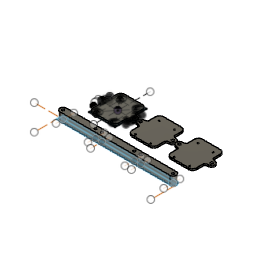
Multi FS40 Bracket v19 (Autodesk Fusion 360 design; units mm, degrees)
Autodesk Fusion 360 part; units mm, degrees
sketch "Schizzo1" plane through (0, 0, 0) normal (0, 0, 1) x (1, 0, 0)
  line L0 (32, -39) -> (-32, -39)
  line L1 (-32, -39) -> (-32, 39)
  line L2 (-32, 39) -> (32, 39)
  line L3 (32, 39) -> (32, -39)
  line L4 (32, -39) -> (-32, 39) construction
  line L5 (-32, -39) -> (32, 39) construction
  line L6 (-19.25, 24.7) -> (19.25, 24.7) construction
  line L7 (19.25, 24.7) -> (19.25, -33.8) construction
  line L8 (19.25, -33.8) -> (-19.25, -33.8) construction
  line L9 (-19.25, -33.8) -> (-19.25, 24.7) construction
  circle A0 centre (-19.25, 24.7) radius 1.7
  line L10 (0, 0) -> (0, 80) construction
  line L11 (0, 0) -> (0, -60) construction
  line L12 (-32, 0) -> (32, 0) construction
  circle A1 centre (-19.25, -33.8) radius 1.7
  circle A2 centre (19.25, -33.8) radius 1.7
  circle A3 centre (19.25, 24.7) radius 1.7
  line L13 (-32, 0) -> (-48, 0) construction
  line L14 (-40, 20.7498) -> (-40, -19.8726) construction
  circle A4 centre (-40, 0) radius 8
  line L15 (-40, -8) -> (-46, -8) construction
  line L16 (-46, -11.1) -> (-32, -11.1) construction
  arc A5 (-32, -11.1) -> (-40, -8) centre (-40, -19.8726) ccw
  arc A6 (-40, 8) -> (-32, 11.1) centre (-40, 19.8726) ccw
  circle A7 centre (40, 0) radius 8
  arc A8 (32, 11.1) -> (40, 8) centre (40, 19.8726) ccw
  arc A9 (40, -8) -> (32, -11.1) centre (40, -19.8726) ccw
  line L17 (-56.7434, -78.6442) -> (226.9, -78.6442)
  line L18 (226.9, -78.6442) -> (226.9, -94.6442)
  line L19 (226.9, -94.6442) -> (-56.7434, -94.6442)
  line L20 (-56.7434, -94.6442) -> (-56.7434, -78.6442)
  circle A10 centre (-48.7434, -86.6442) radius 8
  line L21 (-48.7434, -60) -> (-48.7434, -104.1406) construction
  circle A11 centre (-48.7434, -86.6442) radius 2.9
  line L22 (31.2566, -65) -> (31.2566, -105) construction
  line L23 (226.9, -86.6442) -> (-120, -86.6442) construction
  circle A12 centre (31.2566, -86.6442) radius 2.9
  line L24 (47.4566, -68.4362) -> (47.4566, -114.7306) construction
  circle A13 centre (47.4566, -86.6442) radius 2.9
  line L25 (127.4566, -70) -> (127.4566, -110) construction
  circle A14 centre (127.4566, -86.6442) radius 2.9
  line L26 (143.6566, -70) -> (143.6566, -110) construction
  line L27 (223.6566, -70) -> (223.6566, -110) construction
  circle A15 centre (143.6566, -86.6442) radius 2.9
  circle A16 centre (223.6566, -86.6442) radius 2.9
  circle A17 centre (223.6566, -86.6442) radius 8
  line L28 (-56.7434, -86.6442) -> (231.6566, -86.6442)
  line L29 (231.6566, -86.6442) -> (-56.7434, -86.6442)
  line L30 (-56.7434, -86.6442) -> (-56.7434, -150) construction
  line L31 (231.6566, -86.6442) -> (231.6566, -150) construction
  circle A18 centre (-40, 0) radius 3.1
  circle A19 centre (40, 0) radius 3.1
  circle A20 centre (-22, -29) radius 10
  circle A21 centre (22, -29) radius 10
  circle A22 centre (-22, 29) radius 10
  circle A23 centre (22, 29) radius 10
  dimension "d1" = 64
  dimension "d2" = 78
  dimension "d3" = 33.8
  dimension "d5" = 58.5
  dimension "d6" = 19.25
  dimension "d7" = 38.5
  dimension "d8" = 3.4
  dimension "d9" = 3.4
  dimension "d17" = 8
  dimension "d18" = 16
  dimension "d19" = 3.1
  dimension "d20" = 80
  dimension "d21" = 16
  dimension "d22" = 8
  dimension "d23" = 5.8
  dimension "d24" = 80
  dimension "d25" = 5.8
  dimension "d28" = 96.2
  dimension "d29" = 5.8
  dimension "d30" = 80
  dimension "d32" = 5.8
  dimension "d33" = 96.2
  dimension "d34" = 80
  dimension "d35" = 5.8
  dimension "d36" = 5.8
  dimension "d39" = 6.2
  dimension "d87" = 10
  dimension "d88" = 288.4
  constraint horizontal L0
  constraint perpendicular L0 L1
  constraint parallel L0 L2
  constraint parallel L1 L3
  constraint coincident L4 L10.start
  constraint coincident L5 L10.start
  constraint coincident L10.start L11.start
  constraint horizontal L6
  constraint vertical L7
  constraint horizontal L8
  constraint vertical L9
  constraint coincident L6.start L9.end
  constraint perpendicular L2 L10
  constraint perpendicular L0 L11
  constraint midpoint L1 L12.start
  constraint midpoint L3 L12.end
  constraint coincident L8.end L9.start
  constraint symmetric A0 L11 A3
  constraint symmetric L11 A1 A2
  constraint perpendicular L1 L13
  constraint vertical L14
  constraint coincident A4 L15.start
  constraint coincident L14 L15.start
  constraint tangent A4 L15
  constraint horizontal L16
  constraint coincident L1 L16.end
  constraint coincident L14 A5.centre
  constraint symmetric L13 L15.start A6.start
  constraint symmetric L13 L16.end A6.end
  constraint symmetric L13 A5 A6
  constraint symmetric L10 A4 A7
  constraint symmetric L10 L15.start A9.start
  constraint symmetric L10 L16.end A9.end
  constraint symmetric L10 A5 A9
  constraint symmetric L10 A6.end A8.start
  constraint symmetric L10 A6.start A8.end
  constraint symmetric L10 A6 A8
  constraint horizontal L17
  constraint vertical L18
  constraint horizontal L19
  constraint vertical L20
  constraint tangent L20 A10
  constraint tangent L19 A10
  constraint perpendicular L17 L21
  constraint coincident A10.centre L21
  constraint concentric A10 A11
  constraint perpendicular L19 L22
  constraint midpoint L18 L23.start
  constraint perpendicular L21 L23
  constraint coincident L22 A12.centre
  constraint coincident L23 A12.centre
  constraint perpendicular L19 L24
  constraint coincident L24 A13.centre
  constraint coincident L23 A13.centre
  constraint perpendicular L19 L25
  constraint coincident L25 A14.centre
  constraint coincident L23 A14.centre
  constraint perpendicular L19 L26
  constraint perpendicular L19 L27
  constraint coincident L26 A15.centre
  constraint coincident L23 A15.centre
  constraint coincident L27 A16.centre
  constraint coincident L23 A16.centre
  constraint concentric A16 A17
  constraint tangent L17 A17
  constraint midpoint L20 L28.start
  constraint coincident A17 L28.end
  constraint coincident L23 L28.end
  constraint tangent A10 L30
  constraint perpendicular L28 L30
  constraint tangent A17 L31
  constraint coincident L14.end A5.centre
  constraint coincident L13 A4.centre
  constraint concentric A4 A18
  constraint symmetric L10 A18 A19
  constraint tangent L1 A20
  constraint tangent L0 A20
  constraint symmetric L11 A20 A21
  constraint symmetric L12 A20 A22
  constraint symmetric L12 A21 A23
  measures "d1" distance of L1.end L2.end
  measures "d2" distance of L0.end L1.end
  measures "d3" distance of L10.start L8
  measures "d5" distance of L6 L8
  measures "d6" distance of L10.start L9
  measures "d7" distance of L7 L9
  measures "d8" diameter of A0
  measures "d9" diameter of A1
  measures "d17" distance of L1 L14.start
  measures "d18" diameter of A4
  measures "d19" distance of L15 L16
  measures "d20" distance of L14 A7.centre
  measures "d21" distance of L17.start L19.end
  measures "d22" radius of A10
  measures "d23" diameter of A11
  measures "d24" distance of L21 L22
  measures "d25" diameter of A12
  measures "d28" distance of A10.centre L24
  measures "d29" diameter of A13
  measures "d30" distance of L24 L25
  measures "d32" diameter of A14
  measures "d33" distance of L24 L26.end
  measures "d34" distance of L26 L27
  measures "d35" diameter of A15
  measures "d36" diameter of A16
  measures "d39" diameter of A18
  measures "d87" radius of A20
  measures "d88" distance of L30 L31
extrude "Estrusione1" add sketch "Schizzo1" along normal blind 4 contours L0 L1 L2 L3 A20 A21 A22 A23 | A21 | A20 | L3 A7 A9 | L3 A7 A8 | A7 | L1 A4 A5 | L1 A4 A6 | A4 | A23 | A22 makes body 1
pattern_linear "Serie R1" count 1 spacing 0 along (0, 1, 0) count 3 spacing 96.2 along (1, 0, 0) of bodies 1 makes body 2 at (102.3333, 0.3426, 0) makes body 3 at (198.5333, 0.3426, 0)
extrude "Estrusione2" add sketch "Schizzo1" along normal blind 20 separate body contours L17 A10 A12 A13 A14 A15 A17 L28 L29 | A10 A11 L28 L29 | A10 A11 L28 L29 | L18 A16 A17 L28 L29 | L19 A10 A12 A13 A14 A15 A17 L28 L29 | L18 A17 L28 L29 | L18 A16 A17 L28 L29 | L18 A17 L28 L29 makes body 4
sketch "Schizzo2" plane through (0, 0, 0) normal (0, 0, 1) x (1, 0, 0)
  line L0 (-157.1405, -8.0769) -> (-137.1405, -8.0769)
  line L1 (-137.1405, -8.0769) -> (-137.1405, -3.6769)
  line L2 (-137.1405, -3.6769) -> (-157.1405, -3.6769)
  line L3 (-157.1405, -3.6769) -> (-157.1405, -8.0769)
  line L4 (-157.1405, -5.8769) -> (-137.1405, -5.8769) construction
  line L5 (-147.1405, -3.6769) -> (-147.1405, -8.0769) construction
  line L6 (-141.6405, -8.0769) -> (-152.6405, -8.0769)
  line L7 (-152.6405, -8.0769) -> (-152.6405, -3.6769)
  line L8 (-152.6405, -3.6769) -> (-141.6405, -3.6769)
  line L9 (-141.6405, -3.6769) -> (-141.6405, -8.0769)
  line L10 (-141.6405, -8.0769) -> (-152.6405, -3.6769) construction
  line L11 (-152.6405, -8.0769) -> (-141.6405, -3.6769) construction
  line L12 (-141.6405, -6.6769) -> (-152.6405, -6.6769)
  line L13 (-152.6405, -6.6769) -> (-152.6405, -5.0769)
  line L14 (-152.6405, -5.0769) -> (-141.6405, -5.0769)
  line L15 (-141.6405, -5.0769) -> (-141.6405, -6.6769)
  line L16 (-141.6405, -6.6769) -> (-152.6405, -5.0769) construction
  line L17 (-152.6405, -6.6769) -> (-141.6405, -5.0769) construction
  line L18 (-157.1405, 2.1231) -> (-45.1405, 2.1231)
  line L19 (-45.1405, 2.1231) -> (-45.1405, -13.8769)
  line L20 (-45.1405, -13.8769) -> (-157.1405, -13.8769)
  line L21 (-157.1405, -13.8769) -> (-157.1405, 2.1231)
  line L22 (-101.1405, 2.1231) -> (-101.1405, -35) construction
  line L23 (-49.6405, -3.6769) -> (-60.6405, -3.6769)
  line L24 (-60.6405, -3.6769) -> (-60.6405, -8.0769)
  line L25 (-49.6405, -5.0769) -> (-60.6405, -5.0769)
  line L26 (-49.6405, -8.0769) -> (-49.6405, -3.6769)
  line L27 (-60.6405, -6.6769) -> (-49.6405, -6.6769)
  line L28 (-60.6405, -8.0769) -> (-49.6405, -8.0769)
  line L29 (-152.6405, -5.8769) -> (-36.8883, -5.8769) construction
  line L30 (-96.1405, 2.1231) -> (-96.1405, -17) construction
  circle A0 centre (-96.1405, -5.8769) radius 5
  point P0 (-147.1405, -5.8769)
  point P1 (-147.1405, -5.8769)
  dimension "d40" = 20
  dimension "d41" = 4.4
  dimension "d42" = 11
  dimension "d43" = 4.4
  dimension "d44" = 11
  dimension "d45" = 1.6
  dimension "d50" = 112
  dimension "d51" = 8
  dimension "d52" = 16
  dimension "d69" = 103
  dimension "d70" = 1.4
  dimension "d74" = 5
  constraint horizontal L0
  constraint vertical L1
  constraint horizontal L2
  constraint vertical L3
  constraint midpoint L3 L4.start
  constraint midpoint L1 L4.end
  constraint midpoint L2 L5.start
  constraint midpoint L0 L5.end
  constraint horizontal L6
  constraint perpendicular L6 L7
  constraint parallel L6 L8
  constraint parallel L7 L9
  constraint coincident L10 P1
  constraint coincident L11 P1
  constraint midpoint L5 P1
  constraint horizontal L12
  constraint perpendicular L12 L13
  constraint parallel L12 L14
  constraint parallel L13 L15
  constraint coincident L16 P1
  constraint coincident L17 P1
  constraint coincident P1 P0
  constraint horizontal L18
  constraint vertical L19
  constraint horizontal L20
  constraint vertical L21
  constraint collinear L3 L21
  constraint midpoint L18 L22.start
  constraint perpendicular L20 L22
  constraint symmetric L6.start L22 L24.end
  constraint symmetric L6.end L22 L26.start
  constraint symmetric L7.end L22 L23.start
  constraint symmetric L8.end L22 L23.end
  constraint symmetric L12.start L22 L27.start
  constraint symmetric L12.end L22 L27.end
  constraint symmetric L13.end L22 L25.start
  constraint symmetric L14.end L22 L25.end
  constraint midpoint L7 L29.start
  constraint perpendicular L1 L29
  constraint perpendicular L18 L30
  constraint coincident L18 L30.start
  constraint coincident L30 A0.centre
  constraint coincident L29 A0.centre
  constraint tangent L22 A0
  measures "d40" distance of L1 L3
  measures "d41" distance of L0 L2
  measures "d42" distance of L7.end L8.end
  measures "d43" distance of L6.end L7.end
  measures "d44" distance of L13.end L14.end
  measures "d45" distance of L12.end L13.end
  measures "d50" distance of L19 L21
  measures "d51" distance of L4.start L18.start
  measures "d52" distance of L18 L20
  measures "d69" distance of L7 L26
  measures "d70" distance of L8.end L14
  measures "d74" distance of L22 L30
extrude "Estrusione3" add sketch "Schizzo2" along normal blind 3 separate body contours L0 L6 L7 L9 L12 | L2 L7 L8 L9 L14 | L23 L24 L25 L26 | L24 L26 L27 L28 makes body 5 at (-148.9738, -8.0769, 1) makes body 6 at (-145.3071, -3.6769, 1) makes body 7 at (-56.9738, -8.0769, 1) makes body 8 at (-53.3071, -5.0769, 1)
extrude "Estrusione4" add sketch "Schizzo2" against normal blind 20 separate body contours L0 L2 L3 L7 L13 L21 | L0 L1 L2 L6 L8 L18 L19 L20 L21 | L0 L6 L7 L9 L12 | L0 L1 L2 L9 L15 | L7 L9 L12 L13 L14 L15 | L2 L7 L8 L9 L14 | L23 L24 L25 L26 | L24 L25 L26 L27 | L24 L26 L27 L28 | A0 makes body 9
combine "Combina1" operation add target body 6 tool bodies 9
combine "Combina2" operation add target body 5 tool bodies 6
sketch "Schizzo3" plane through (-152.6405, 0, 0) normal (-1, 0, 0) x (0, -1, 0)
  line L0 (3.6769, 0) -> (5.0769, 0)
  line L1 (5.0769, 0) -> (5.0769, 3)
  line L2 (5.0769, 3) -> (3.6769, 3)
  line L3 (3.6769, 3) -> (3.6769, 0)
sketch "Schizzo5" plane through (-152.6405, -5.3769, 2.25) normal (-1, 0, 0) x (0, -1, 0)
  line L0 (0, 0.7406) -> (0, 4.484) construction
  line L1 (1, 0.7406) -> (1, 4.4786) construction
  line L2 (0, 0.7406) -> (1, 0.7406) construction
  line L3 (0.5, 0.7406) -> (0.5, 3.1) construction
  line L4 (0, 0.7406) -> (-2.9121, 0.7406) construction
  line L5 (0, 0.7406) -> (-2.2, 0.7406)
  line L6 (0, 0.7406) -> (0, 3.2406)
  line L7 (0, 3.2406) -> (-2.2, 0.7406)
  line L8 (1, 3.2406) -> (3.2, 0.7406)
  line L9 (1, 0.7406) -> (3.2, 0.7406)
  line L10 (1, 0.7406) -> (1, 3.2406)
  dimension "d59" = 2.2
  dimension "d60" = 2.5
  dimension "d63" = 1
  constraint vertical L0
  constraint vertical L1
  constraint midpoint L2 L3.start
  constraint perpendicular L2 L3
  constraint perpendicular L0 L4
  constraint perpendicular L0 L5
  constraint coincident L0 L6.end
  constraint symmetric L0.start L3 L1.start
  constraint symmetric L3 L5.end L8.end
  constraint symmetric L3 L6.end L8.start
  measures "d59" distance of L0.start L5.end
  measures "d60" distance of L2 L6.end
  measures "d63" distance of L0 L10
extrude "Estrusione6" add sketch "Schizzo5" against normal blind 11 bodies 5
sketch "Schizzo6" plane through (-49.6405, 0, 0) normal (1, 0, 0) x (0, 1, 0)
  line L0 (-5.0769, 0) -> (-3.6769, 0)
  line L1 (-3.6769, 0) -> (-3.6769, 3)
  line L2 (-3.6769, 3) -> (-5.0769, 3)
  line L3 (-5.0769, 3) -> (-5.0769, 0)
  line L4 (-6.0769, 3) -> (-5.0769, 3) construction
  line L5 (-5.5769, 3) -> (-5.5769, 6.3) construction
  line L6 (-6.0769, 3) -> (-8.2769, 3)
  line L7 (-6.0769, 3) -> (-6.0769, 5.5)
  line L8 (-6.0769, 5.5) -> (-8.2769, 3)
  line L9 (-5.0769, 5.5) -> (-2.8769, 3)
  line L10 (-5.0769, 3) -> (-5.0769, 5.5)
  line L11 (-5.0769, 3) -> (-2.8769, 3)
  dimension "d64" = 1
  dimension "d65" = 2.2
  dimension "d66" = 2.5
  constraint horizontal L4
  constraint midpoint L4 L5.start
  constraint perpendicular L4 L5
  constraint parallel L4 L6
  constraint perpendicular L4 L7
  constraint symmetric L4.start L5 L2.end
  constraint symmetric L5 L6.end L9.end
  constraint symmetric L5 L7.end L9.start
  constraint collinear L2 L11
  constraint collinear L3 L10
  measures "d64" distance of L4.start L2.end
  measures "d65" distance of L6.end L7
  measures "d66" distance of L4.start L7.end
extrude "Estrusione7" add sketch "Schizzo6" against normal blind 11 separate body contours L2 L9 L10 L11 | L6 L7 L8 makes body 10 at (-53.3071, -6.8102, 4.6667) makes body 11 at (-56.9738, -4.3436, 4.6667)
combine "Combina5" operation add target body 7 tool bodies 8 11 5
combine "Combina7" operation add target body 7 tool bodies 10
sketch "Schizzo7" plane through (-45.1405, 0, 0) normal (1, 0, 0) x (0, 1, 0)
  line L0 (2.1231, 0) -> (-13.8769, 0)
  line L1 (-13.8769, 0) -> (-13.8769, -20)
  line L2 (-13.8769, -20) -> (2.1231, -20)
  line L3 (2.1231, -20) -> (2.1231, 0)
  line L4 (-5.8769, 0) -> (-5.8769, -20) construction
  line L5 (-13.8769, -10) -> (2.1231, -10) construction
  circle A0 centre (-5.8769, -10) radius 4
  dimension "d71" = 8
  constraint midpoint L0 L4.start
  constraint midpoint L2 L4.end
  constraint midpoint L1 L5.start
  constraint midpoint L3 L5.end
  constraint midpoint L5 A0.centre
  measures "d71" diameter of A0
extrude "Estrusione8" cut sketch "Schizzo7" against normal blind 51 contours A0 bodies 7
extrude "Estrusione9" cut sketch "Schizzo2" against normal blind 14 contours A0 bodies 7
sketch "Schizzo8" plane through (0, -13.8769, 0) normal (0, -1, 0) x (1, 0, 0)
  line L0 (-45.1405, 0) -> (-157.1405, 0)
  line L1 (-157.1405, 0) -> (-157.1405, -20)
  line L2 (-157.1405, -20) -> (-45.1405, -20)
  line L3 (-45.1405, -20) -> (-45.1405, 0)
  line L4 (-157.1405, -10) -> (-45.1405, -10) construction
  line L5 (-67, -5) -> (-63, -5)
  line L6 (-63, -5) -> (-63, -15)
  line L7 (-63, -15) -> (-67, -15)
  line L8 (-67, -15) -> (-67, -5)
  line L9 (-67, 6) -> (-67, -24) construction
  line L10 (-67, -10) -> (-63, -10) construction
  line L11 (-67, -7) -> (-63, -7)
  line L12 (-67, -13) -> (-63, -13)
  dimension "d80" = 4
  dimension "d81" = 10
  dimension "d82" = 2
  constraint midpoint L1 L4.start
  constraint midpoint L3 L4.end
  constraint horizontal L5
  constraint vertical L6
  constraint horizontal L7
  constraint vertical L8
  constraint perpendicular L2 L9
  constraint midpoint L8 L10.start
  constraint midpoint L6 L10.end
  constraint collinear L4 L10
  constraint collinear L8 L9
  constraint coincident L9 L11.start
  constraint coincident L6 L11.end
  constraint perpendicular L6 L11
  constraint symmetric L4 L11.start L12.start
  constraint symmetric L4 L11.end L12.end
  measures "d80" distance of L5.start L5.end
  measures "d81" distance of L5.start L7
  measures "d82" distance of L5 L11
extrude "Estrusione10" cut sketch "Schizzo8" against normal blind 8 contours L6 L8 L11 L12 bodies 7
extrude "Estrusione11" cut sketch "Schizzo8" against normal blind 16 contours L5 L6 L8 L11 | L6 L7 L8 L12 bodies 7
hidden bodies 7
equation "d6 = 38.50 mm / 2"
equation "d72 = ( ( -112 / 2 ) * 1 mm ) + 5 mm"
named bodies: "Basetta 1", "Basetta 2", "Basetta 3", "Trave", "Fissaggio Lampada"
